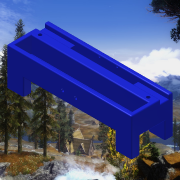
# Autodesk Inventor part: C30_ZP_Solenoid Holder
Saved by Autodesk Inventor 2015 SP1 (Build 190203100, 203)
## iProperties
Created: 2016-01-30
Part Number: C30_ZP_Solenoid Holder
Material: Generic
Document SubType Name: Modeling
Designer: Administrator
Density: 1 g/cm^3
Appearance: Blue - Wall Paint - Glossy
Mass: 257.88 g
Surface Area: 656.414 cm^2
Volume: 257.88 cm^3
Author: Administrator
Autodesk Inventor part; units mm, degrees
ref_plane "YZ Plane" through (0, 0, 0) normal (1, 0, 0) x (0, 1, 0)
ref_plane "XZ Plane" through (0, 0, 0) normal (0, 1, 0) x (-1, 0, 0)
ref_plane "XY Plane" through (0, 0, 0) normal (0, 0, 1) x (1, 0, 0)
sketch "Sketch1" plane through (0, 0, 0) normal (0, 0, 1) x (1, 0, 0)
  line L0 (0, 0) -> (190.5, 0)
  line L1 (190.5, 0) -> (190.5, 31.75)
  line L2 (190.5, 31.75) -> (0, 31.75)
  line L3 (0, 31.75) -> (0, 0)
  dimension "d0" = 190.5
  dimension "d1" = 31.75
  dimension "d2" = 190.5
  constraints: 8 end point, 2 perpendicular, 1 horizontal
  measures "d0" distance of L0.start L0.end
  measures "d1" distance of L0.end L1.end
  measures "d2" distance of L1.end L2.end
extrude "Extrusion1" add sketch "Sketch1" along normal blind 63.5
sketch "Sketch3" plane through (0, 0, 0) normal (0, -1, 0) x (1, 0, 0)
  line L0 (0, 0) -> (25.4, 0)
  line L1 (25.4, 0) -> (25.4, 12.7)
  line L2 (25.4, 12.7) -> (0, 12.7)
  line L3 (0, 12.7) -> (0, 0)
  line L4 (0, 63.5) -> (25.4, 63.5)
  line L5 (25.4, 63.5) -> (25.4, 50.8)
  line L6 (25.4, 50.8) -> (0, 50.8)
  line L7 (0, 50.8) -> (0, 63.5)
  line L8 (190.5, 63.5) -> (165.1, 63.5)
  line L9 (165.1, 63.5) -> (165.1, 50.8)
  line L10 (165.1, 50.8) -> (190.5, 50.8)
  line L11 (190.5, 50.8) -> (190.5, 63.5)
  line L12 (190.5, 0) -> (165.1, 0)
  line L13 (165.1, 0) -> (165.1, 12.7)
  line L14 (165.1, 12.7) -> (190.5, 12.7)
  line L15 (190.5, 12.7) -> (190.5, 0)
  dimension "d5" = 25.4
  dimension "d6" = 25.4
  dimension "d7" = 25.4
  dimension "d8" = 25.4
  dimension "d9" = 12.7
  dimension "d10" = 12.7
  dimension "d11" = 12.7
  dimension "d12" = 12.7
  constraints: 32 end point, 8 parallel, 4 horizontal, 4 perpendicular
  measures "d5" distance of L2.end L1.end
  measures "d6" distance of L5.end L6.end
  measures "d7" distance of L10.end L9.end
  measures "d8" distance of L13.end L14.end
  measures "d9" distance between parallel lines of L4 L6
  measures "d10" distance between parallel lines of L0 L2
  measures "d11" distance between parallel lines of L8 L10
  measures "d12" distance between parallel lines of L12 L14
extrude "Extrusion2" add sketch "Sketch3" along normal blind 25.4
sketch "Sketch4" plane through (0, 31.75, 0) normal (0, 1, 0) x (1, 0, 0)
  line L0 (46.99, -6.35) -> (143.51, -6.35)
  line L1 (143.51, -6.35) -> (143.51, -19.05)
  line L2 (143.51, -19.05) -> (46.99, -19.05)
  line L3 (46.99, -19.05) -> (46.99, -6.35)
  line L4 (0, 0) -> (0, -63.5) projected
  line L5 (25.4, 0) -> (165.1, 0) projected
  dimension "d15" = 96.52
  dimension "d16" = 46.99
  dimension "d28" = 12.7
  dimension "d50" = 6.35
  constraints: 8 end point, 2 parallel, 1 horizontal, 1 perpendicular
  measures "d15" distance of L1.end L2.end
  measures "d16" distance between parallel lines of L4 L3
  measures "d28" distance between parallel lines of L2 L0
  measures "d50" distance between parallel lines of L5 L0
extrude "Extrusion3" cut sketch "Sketch4" against normal blind 25.4
sketch "Sketch5" plane through (0, 6.35, 0) normal (0, 1, 0) x (1, 0, 0)
  line L0 (46.99, -6.35) -> (143.51, -6.35) projected
  line L1 (190.5, 0) -> (190.5, -63.5) projected
  line L2 (46.99, -6.35) -> (143.51, -6.35) projected
  line L3 (143.51, -19.05) -> (46.99, -19.05) projected
  line L4 (92.075, -6.35) -> (111.125, -6.35)
  line L5 (111.125, -6.35) -> (111.125, -19.05)
  line L6 (111.125, -19.05) -> (92.075, -19.05)
  line L7 (92.075, -19.05) -> (92.075, -6.35)
  point P0 (0, 0)
  dimension "d29" = 19.05
  dimension "d30" = 79.375
  constraints: 8 end point, 2 parallel, 2 point on line, 1 horizontal, 1 perpendicular
  measures "d29" distance between parallel lines of L5 L7
  measures "d30" distance between parallel lines of L1 L5
extrude "Extrusion4" cut sketch "Sketch5" against normal blind 25.4
sketch "Sketch6" plane through (0, 31.75, 0) normal (0, 1, 0) x (1, 0, 0)
  line L0 (6.35, -31.75) -> (184.15, -31.75)
  line L1 (184.15, -31.75) -> (184.15, -57.15)
  line L2 (184.15, -57.15) -> (6.35, -57.15)
  line L3 (6.35, -57.15) -> (6.35, -31.75)
  line L4 (0, 0) -> (0, -63.5) projected
  line L5 (190.5, -63.5) -> (0, -63.5) projected
  dimension "d24" = 177.8
  dimension "d40" = 25.4
  dimension "d41" = 6.35
  dimension "d42" = 6.35
  constraints: 8 end point, 2 parallel, 1 horizontal, 1 perpendicular
  measures "d24" distance of L1.end L2.end
  measures "d40" distance of L2.end L0.start
  measures "d41" distance between parallel lines of L4 L3
  measures "d42" distance between parallel lines of L5 L2
extrude "Extrusion5" cut sketch "Sketch6" against normal blind 25.4
sketch "Sketch8" plane through (0, 6.35, 0) normal (0, 1, 0) x (1, 0, 0)
  line L0 (87.3125, -37.1094) -> (115.8875, -37.1094)
  line L1 (115.8875, -37.1094) -> (115.8875, -50.4444)
  line L2 (115.8875, -50.4444) -> (87.3125, -50.4444)
  line L3 (87.3125, -50.4444) -> (87.3125, -37.1094)
  line L4 (190.5, 0) -> (190.5, -63.5) projected
  line L5 (6.35, -31.75) -> (184.15, -31.75) projected
  point P0 (0, 0)
  point P1 (184.15, -31.75)
  point P2 (190.5, -39.1543)
  dimension "d34" = 13.335
  dimension "d35" = 28.575
  dimension "d36" = 74.6125
  dimension "d37" = 5.3594
  constraints: 8 end point, 2 parallel, 1 horizontal, 1 perpendicular, 1 other
  measures "d34" distance of L2.end L0.start
  measures "d35" distance of L1.end L2.end
  measures "d36" distance between parallel lines of L4 L1
extrude "Extrusion6" cut sketch "Sketch8" against normal blind 25.4
sketch "Sketch9" plane through (0, 0, 63.5) normal (0, 0, 1) x (1, 0, 0)
  point P0 (0, 0)
sketch "Sketch10" plane through (0, 0, 63.5) normal (0, 0, 1) x (1, 0, 0)
  line L0 (120.25, 41.35) -> (117.25, 41.35) projected
  line L1 (117.25, 37.85) -> (117.25, 41.35) projected
  line L2 (111.25, 37.85) -> (117.25, 37.85) projected
  line L3 (111.25, 37.85) -> (111.25, 41.35) projected
  line L4 (111.25, 41.35) -> (70.25, 41.35) projected
  line L5 (70.25, 41.35) -> (70.25, 6.35) projected
  line L6 (70.25, 6.35) -> (120.25, 6.35) projected
  line L7 (120.25, 6.35) -> (120.25, 41.35) projected
  circle A0 centre (85.25, 13.35) radius 2.15 projected
  circle A1 centre (105.25, 13.35) radius 2.15 projected
  point P0 (0, 0)
hole "Hole1" at (85.25, 13.35, 63.5) at (105.25, 13.35, 63.5) direction (0, 0, -1) diameter 4.3 end up to surface
sketch "Sketch11" plane through (0, 0, 0) normal (0, 0, -1) x (-1, 0, 0)
  circle A0 centre (-83.9725, 28.95) radius 1.6 projected
  circle A1 centre (-110.9725, 28.95) radius 1.6 projected
  line L0 (-118.4725, 33.05) -> (-118.4725, 6.35) projected
  line L1 (-76.4725, 6.35) -> (-118.4725, 6.35) projected
  line L2 (-76.4725, 6.35) -> (-76.4725, 33.05) projected
  line L3 (-76.4725, 33.05) -> (-118.4725, 33.05) projected
  point P0 (0, 0)
hole "Hole2" at (83.9725, 28.95, 0) at (110.9725, 28.95, 0) direction (0, 0, 1) diameter 3.2 depth 12.7 tip angle 118
sketch "Sketch12" plane through (190.5, 31.75, 63.5) normal (1, 0, 0) x (0, 0, -1)
  line L0 (57.15, 0) -> (57.15, -25.4) projected
  line L1 (44.45, 0) -> (57.15, 0)
  line L2 (57.15, 0) -> (57.15, -6.35)
  line L3 (57.15, -6.35) -> (44.45, -6.35)
  line L4 (44.45, -6.35) -> (44.45, 0)
  point P0 (63.5, -31.75)
  dimension "d58" = 6.35
  constraints: 8 end point, 2 parallel, 1 horizontal, 1 perpendicular, 1 point on line
  measures "d58" distance between parallel lines of L1 L3
extrude "Extrusion7" cut sketch "Sketch12" against normal blind 190.5
sketch "Sketch13" plane through (0, 31.75, 63.5) normal (0, 1, 0) x (1, 0, 0)
  line L0 (6.35, 6.35) -> (6.35, 31.75) projected
  line L1 (6.35, 31.75) -> (184.15, 31.75) projected
  line L2 (184.15, 31.75) -> (184.15, 6.35) projected
  line L3 (184.15, 6.35) -> (6.35, 6.35) projected
  line L4 (190.5, 44.45) -> (0, 44.45) projected
  line L5 (0, 44.45) -> (0, 0) projected
  line L6 (190.5, 0) -> (0, 0) projected
  line L7 (190.5, 44.45) -> (190.5, 0) projected
  point P0 (190.5, 0)
  point P1 (12.7, 38.1)
  point P2 (177.8, 38.1)
  dimension "d74" = 12.7
  dimension "d75" = 6.35
  dimension "d76" = 12.7
  dimension "d77" = 6.35
  measures "d74" distance from line of L7 point (177.8, 38.1)
  measures "d75" distance from line of L4 point (177.8, 38.1)
  measures "d76" distance from line of L5 point (12.7, 38.1)
  measures "d77" distance from line of L4 point (12.7, 38.1)
hole "Hole3" at (12.7, 31.75, 25.4) at (177.8, 31.75, 25.4) direction (0, -1, 0) diameter 5.1054 end through all clearance for "Flat Head Machine Screw (82)" size "#10" standard "Ansi Unified Screw Threads"
fillet "Fillet1" radius 1.5875 38 edges at (165.1, -12.7, 63.5) (95.25, 0, 63.5) (25.4, -12.7, 63.5) (0, 3.175, 63.5) (0, -12.7, 50.8) (25.4, -12.7, 50.8) (0, 3.175, 0) (0, -12.7, 12.7) (0, 0, 31.75) (25.4, -12.7, 0) (25.4, -12.7, 12.7) (95.25, 0, 0) (165.1, -12.7, 0) (165.1, -12.7, 50.8) (190.5, 3.175, 63.5) (190.5, -12.7, 50.8) (190.5, 0, 31.75) (190.5, -12.7, 12.7) (190.5, 3.175, 0) (165.1, -12.7, 12.7) (95.25, 31.75, 63.5) (190.5, 31.75, 41.275) (190.5, 31.75, 3.175) (190.5, 25.4, 12.7) (190.5, 28.575, 19.05) (95.25, 31.75, 0) (0, 31.75, 3.175) (0, 28.575, 6.35) (0, 25.4, 12.7) (0, 28.575, 19.05) (0, 31.75, 41.275) (190.5, 28.575, 6.35) (6.35, 31.75, 44.45) (95.25, 31.75, 31.75) (95.25, 31.75, 57.15) (184.15, 31.75, 44.45) (95.25, 31.75, 6.35) (95.25, 31.75, 19.05)
body "Solid1"
